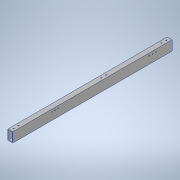
# Autodesk Inventor part: オムニ_角柱3
Saved by Autodesk Inventor 2021 (Build 250183000, 183)
## iProperties
Created: 2021-12-02
Part Number: オムニ_角柱3
Material: アルミニウム 6061
Document SubType Name: Modeling
Designer: 堀川皓史
Density: 2.7 g/cm^3
Appearance: アルミニウム - フラット
Mass: 216.625 g
Surface Area: 807.202 cm^2
Volume: 80.2313 cm^3
Author: 堀川皓史
Autodesk Inventor part; units mm, degrees
ref_plane "YZ Plane" through (0, 0, 0) normal (1, 0, 0) x (0, 1, 0)
ref_plane "XZ Plane" through (0, 0, 0) normal (0, 1, 0) x (-1, 0, 0)
ref_plane "XY Plane" through (0, 0, 0) normal (0, 0, 1) x (1, 0, 0)
sketch "スケッチ1" plane through (0, 0, 0) normal (0, 0, 1) x (1, 0, 0)
  line L0 (7.5, 15) -> (-7.5, 15)
  line L1 (-7.5, 15) -> (-7.5, -15)
  line L2 (-7.5, -15) -> (7.5, -15)
  line L3 (7.5, -15) -> (7.5, 15)
  line L4 (7.5, 15) -> (-7.5, -15) construction
  line L5 (-7.5, 15) -> (7.5, -15) construction
  line L6 (-5.5, 13) -> (5.5, 13)
  line L7 (5.5, 13) -> (5.5, -13)
  line L8 (5.5, -13) -> (-5.5, -13)
  line L9 (-5.5, -13) -> (-5.5, 13)
  point P0 (0, 0)
  dimension "d0" = 15
  dimension "d1" = 30
  dimension "d2" = 2
  constraints: 20 end point, 4 parallel, 2 midpoint, 2 perpendicular, 1 horizontal, 3 other
  measures "d0" distance of L2.end L1.end
  measures "d1" distance of L1.end L0.end
  measures "d2" distance between parallel lines of L0 L6
extrude "押し出し1" add sketch "スケッチ1" along normal blind 490
sketch "スケッチ2" plane through (-7.5, 15, 0) normal (0, 1, 0) x (1, 0, 0)
  circle A0 centre (7.5, -10) radius 1.6
  circle A1 centre (7.5, -25) radius 1.6
  circle A2 centre (7.5, -480) radius 1.6
  circle A3 centre (7.5, -465) radius 1.6
  line L0 (15, 0) -> (0, 0) projected
  line L1 (15, -490) -> (0, -490) projected
  circle A4 centre (7.5, -195) radius 1.6
  circle A5 centre (7.5, -210) radius 1.6
  point P0 (7.5, 0)
  point P1 (7.5, 0)
  dimension "d5" = 3.2
  dimension "d6" = 3.2
  dimension "d7" = 3.2
  dimension "d8" = 3.2
  dimension "d9" = 10
  dimension "d10" = 15
  dimension "d11" = 10
  dimension "d12" = 15
  dimension "d15" = 3.2
  dimension "d16" = 3.2
  dimension "d17" = 15
  dimension "d18" = 170
  constraints: 6 centre point, 6 vertical alignment, 1 midpoint
  measures "d5" diameter of A0
  measures "d6" diameter of A1
  measures "d7" diameter of A2
  measures "d8" diameter of A3
  measures "d9" distance of point (7.5, 0) A0.centre
  measures "d10" distance of A0.centre A1.centre
  measures "d11" distance from line of A2.centre L1
  measures "d12" distance of A3.centre A2.centre
  measures "d15" diameter of A4
  measures "d16" diameter of A5
  measures "d17" distance of A4.centre A5.centre
  measures "d18" distance of A1.centre A4.centre
extrude "押し出し2" cut sketch "スケッチ2" against normal through all
sketch "スケッチ3" plane through (7.5, -15, 0) normal (1, 0, 0) x (0, 0, -1)
  circle A0 centre (-50, 22.5) radius 1.6
  circle A1 centre (-60, 22.5) radius 1.6
  circle A2 centre (-70, 22.5) radius 1.6
  line L0 (0, 30) -> (-490, 30) projected
  circle A3 centre (-350, 22.5) radius 1.6
  circle A4 centre (-360, 22.5) radius 1.6
  circle A5 centre (-370, 22.5) radius 1.6
  point P0 (0, 15)
  dimension "d19" = 3.2
  dimension "d20" = 3.2
  dimension "d21" = 3.2
  dimension "d22" = 7.5
  dimension "d23" = 50
  dimension "d24" = 10
  dimension "d25" = 10
  dimension "d26" = 3.2
  dimension "d27" = 3.2
  dimension "d28" = 3.2
  dimension "d29" = 10
  dimension "d30" = 10
  dimension "d31" = 300
  constraints: 6 centre point, 5 horizontal alignment
  measures "d19" diameter of A0
  measures "d20" diameter of A1
  measures "d21" diameter of A2
  measures "d22" distance from line of L0 A0.centre
  measures "d23" horizontal distance of A0.centre point (0, 15)
  measures "d24" distance of A0.centre A1.centre
  measures "d25" distance of A1.centre A2.centre
  measures "d26" diameter of A3
  measures "d27" diameter of A4
  measures "d28" diameter of A5
  measures "d29" distance of A3.centre A4.centre
  measures "d30" distance of A4.centre A5.centre
  measures "d31" distance of A1.centre A4.centre
extrude "押し出し3" cut sketch "スケッチ3" against normal through all
